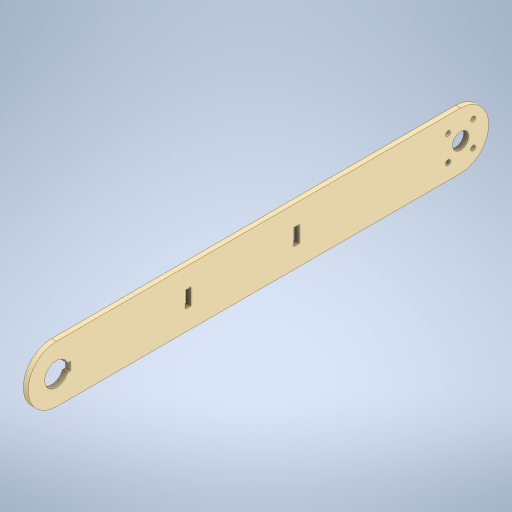
# Autodesk Inventor part: brazo1
Saved by Autodesk Inventor 2024.3 (Build 283343000, 343)
## iProperties
Created: 2024-05-14
Part Number: brazo1
Material: PMMA Plastic
Document SubType Name: Modeling
Designer: USUARIO
Density: 1.188 g/cm^3
Appearance: Beige
Mass: 33.3896 g
Surface Area: 210.718 cm^2
Volume: 28.1058 cm^3
Author: USUARIO
Autodesk Inventor part; units mm, degrees
ref_plane "YZ Plane" through (0, 0, 0) normal (1, 0, 0) x (0, 1, 0)
ref_plane "XZ Plane" through (0, 0, 0) normal (0, 1, 0) x (-1, 0, 0)
ref_plane "XY Plane" through (0, 0, 0) normal (0, 0, 1) x (1, 0, 0)
sketch "Sketch1" plane through (0, 0, 0) normal (1, 0, 0) x (0, 1, 0)
  line L0 (0, 0) -> (0, -250) construction
  circle A0 centre (0, -250) radius 5
  arc A1 (0, -17.5) -> (17.5, 0) centre (0, 0) ccw construction
  arc A2 (0, -232.5) -> (-17.5, -250) centre (0, -250) ccw construction
  line L1 (17.5, 0) -> (17.5, -250)
  line L2 (-17.5, 0) -> (-17.5, -250)
  arc A3 (-17.5, 0) -> (0, -17.5) centre (0, 0) ccw construction
  arc A4 (17.5, 0) -> (-17.5, 0) centre (0, 0) ccw
  arc A5 (17.5, -250) -> (0, -232.5) centre (0, -250) ccw construction
  arc A6 (-17.5, -250) -> (17.5, -250) centre (0, -250) ccw
  line L3 (0, 0) -> (0, -80) construction
  line L4 (0, -80) -> (5, -80) construction
  line L5 (5, -80) -> (5, -83)
  line L6 (5, -83) -> (-5, -83) construction
  line L7 (-5, -83) -> (-5, -80)
  line L8 (-5, -80) -> (0, -80) construction
  line L9 (0, -250) -> (0, -150) construction
  line L10 (0, -150) -> (5, -150) construction
  line L11 (5, -150) -> (5, -147)
  line L12 (5, -147) -> (-5, -147) construction
  line L13 (-5, -147) -> (-5, -150)
  line L14 (0, -150) -> (-5, -150) construction
  line L15 (7.5, 0) -> (7.5, -6) construction
  arc A7 (0, -7.25) -> (2.5, -6.8053) centre (0, 0) ccw construction
  line L16 (0, -7.25) -> (2.5, -7.25) construction
  line L17 (2.5, -7.25) -> (-2.5, -7.25) construction
  line L18 (-2.5, -7.25) -> (-2.5, -8.75)
  line L19 (-2.5, -8.75) -> (2.5, -8.75)
  line L20 (2.5, -8.75) -> (2.5, -7.25)
  line L21 (2.5, -7.25) -> (2.5, -6.8053)
  line L22 (-2.5, -7.25) -> (-2.5, -6.8053)
  arc A8 (-2.5, -6.8053) -> (0, -7.25) centre (0, 0) ccw construction
  arc A9 (2.5, -6.8053) -> (-2.5, -6.8053) centre (0, 0) ccw
  line L23 (0, -250) -> (7.75, -250) construction
  line L24 (7.75, -250) -> (7.75, -257.75) construction
  line L25 (7.75, -257.75) -> (0, -257.75) construction
  line L26 (0, -257.75) -> (0, -250) construction
  line L27 (7.75, -257.75) -> (-7.75, -257.75) construction
  line L28 (-7.75, -257.75) -> (-7.75, -242.25) construction
  line L29 (-7.75, -242.25) -> (7.75, -242.25) construction
  line L30 (7.75, -242.25) -> (7.75, -257.75) construction
  circle A10 centre (7.75, -242.25) radius 1.5
  circle A11 centre (7.75, -257.75) radius 1.5
  circle A12 centre (-7.75, -257.75) radius 1.5
  circle A13 centre (-7.75, -242.25) radius 1.5
  line L31 (5, -80) -> (5, -79.75)
  line L32 (5, -79.75) -> (-5, -79.75)
  line L33 (-5, -79.75) -> (-5, -80)
  line L34 (-5, -83) -> (-5, -83.25)
  line L35 (-5, -83.25) -> (5, -83.25)
  line L36 (5, -83.25) -> (5, -83)
  line L37 (-5, -147) -> (-5, -146.75)
  line L38 (-5, -146.75) -> (5, -146.75)
  line L39 (5, -146.75) -> (5, -147)
  line L40 (5, -150) -> (5, -150.25)
  line L41 (5, -150.25) -> (-5, -150.25)
  line L42 (-5, -150.25) -> (-5, -150)
  dimension "d1" = 250
  dimension "d2" = 10
  dimension "d3" = 35
  dimension "d4" = 35
  dimension "d5" = 80
  dimension "d6" = 5
  dimension "d7" = 3
  dimension "d9" = 100
  dimension "d10" = 3
  dimension "d14" = 10
  dimension "d27" = 2.5
  dimension "d28" = 5
  dimension "d29" = 1.5
  dimension "d30" = 7.25
  dimension "d31" = 7.75
  dimension "d32" = 7.75
  dimension "d33" = 15.5
  dimension "d34" = 15.5
  dimension "d35" = 3
  dimension "d36" = 3
  dimension "d37" = 3
  dimension "d38" = 3
  dimension "d39" = 64
  dimension "d40" = 0.25
  dimension "d41" = 10
  dimension "d42" = 0.25
  dimension "d43" = 0.25
  dimension "d44" = 10
  dimension "d45" = 0.25
  dimension "d46" = 0.25
  dimension "d47" = 10
  dimension "d48" = 0.25
  dimension "d49" = 0.25
  dimension "d50" = 10
  dimension "d51" = 0.25
  constraints: 86 end point, 18 point on circle, 15 perpendicular, 14 centre point, 13 point on line, 9 coincident, 7 parallel, 6 tangent, 5 vertical, 3 horizontal, 1 midpoint
  measures "d1" distance of L0.start L0.end
  measures "d2" diameter of A0
  measures "d3" diameter of A1
  measures "d4" diameter of A2
  measures "d5" distance of L3.start L3.end
  measures "d6" distance of L3.end L4.end
  measures "d7" distance of L4.end L5.end
  measures "d9" distance of L9.start L9.end
  measures "d10" distance of L10.end L11.end
  measures "d14" distance of L5.end L6.end
  measures "d27" distance of L16.start L16.end
  measures "d28" distance of L19.end L18.end
  measures "d29" distance of L18.end L17.end
  measures "d30" radius of A9
  measures "d31" distance of L24.end L25.end
  measures "d32" distance of L23.end L24.end
  measures "d33" distance of L28.end L29.end
  measures "d34" distance of L27.end L28.end
  measures "d35" diameter of A10
  measures "d36" diameter of A11
  measures "d37" diameter of A12
  measures "d38" diameter of A13
  measures "d39" distance between parallel lines of L12 L6
  measures "d40" distance of L4.end L31.end
  measures "d41" distance of L31.end L32.end
  measures "d42" distance of L32.end L7.end
  measures "d43" distance of L6.end L34.end
  measures "d44" distance of L34.end L35.end
  measures "d45" distance of L35.end L5.end
  measures "d46" distance of L12.end L37.end
  measures "d47" distance of L37.end L38.end
  measures "d48" distance of L38.end L11.end
  measures "d49" distance of L10.end L40.end
  measures "d50" distance of L40.end L41.end
  measures "d51" distance of L41.end L13.end
extrude "Extrusion1" add sketch "Sketch1" along normal blind 3
body "Solid1"
